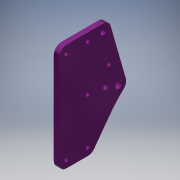
# Autodesk Inventor part: carriage plate square 2
Saved by Autodesk Inventor 2017 SP1 (Build 210196100, 196)
## iProperties
Created: 2018-01-19
Part Number: carriage plate square 2
Material: Aluminum 6061
Document SubType Name: Modeling
Designer: Ben
Density: 2.7 g/cm^3
Appearance: Smooth - Purple
Mass: 147.998 g
Surface Area: 209.147 cm^2
Volume: 54.8139 cm^3
Author: Ben
Autodesk Inventor part; units mm, degrees
ref_plane "YZ Plane" through (0, 0, 0) normal (1, 0, 0) x (0, 1, 0)
ref_plane "XZ Plane" through (0, 0, 0) normal (0, 1, 0) x (-1, 0, 0)
ref_plane "XY Plane" through (0, 0, 0) normal (0, 0, 1) x (1, 0, 0)
sketch "Sketch1" plane through (0, 0, 0) normal (1, 0, 0) x (0, 1, 0)
  line L0 (-420.7503, 12.7) -> (420.7488, 12.7) construction
  line L1 (420.7488, 12.7) -> (420.7488, -12.7) construction
  line L2 (420.7488, -12.7) -> (-420.7503, -12.7) construction
  line L3 (-420.7503, -12.7) -> (-420.7503, 12.7) construction
  line L4 (0, 0) -> (0, -26.6192) construction
  circle A0 centre (0, -26.6192) radius 2.54
  circle A1 centre (38.1, 26.6192) radius 2.54
  circle A2 centre (-76.2, 26.6192) radius 2.54
  line L5 (38.1, 26.6192) -> (-76.2, 26.6192) construction
  line L6 (0, 0) -> (0, 26.6192) construction
  circle A3 centre (0, -26.6192) radius 15.875 construction
  circle A4 centre (38.1, 26.6192) radius 15.875 construction
  circle A5 centre (-76.2, 26.6192) radius 15.875 construction
  line L7 (0, -26.6192) -> (-76.2, 26.6192) construction
  arc A6 (47.625, 26.6192) -> (38.1, 36.1442) centre (38.1, 26.6192) ccw
  arc A7 (-76.2, 36.1442) -> (-85.725, 26.6192) centre (-76.2, 26.6192) ccw
  line L8 (38.1, 36.1442) -> (-76.2, 36.1442)
  line L9 (47.625, 26.6192) -> (47.625, -19.05)
  line L10 (-85.725, 0) -> (-85.725, 26.6192)
  line L11 (-76.2, 26.6192) -> (-76.2, 0) construction
  line L12 (38.1, 26.6192) -> (38.1, 0) construction
  circle A8 centre (38.1, 0) radius 2.667
  circle A9 centre (-76.2, 0) radius 2.667
  line L13 (47.625, 0) -> (-85.725, 0) construction
  line L14 (-85.725, 0) -> (-420.7503, 0) construction
  circle A10 centre (-19.05, 0) radius 2.667
  line L15 (0, -26.6192) -> (38.1, 26.6192) construction
  line L16 (0, -26.6192) -> (0, -52.0192) construction
  line L17 (13.9446, -26.6192) -> (-16.4809, -26.6192) construction
  circle A11 centre (38.1, -19.05) radius 3.302
  circle A12 centre (-22.225, -22.225) radius 3.302
  line L18 (38.1, -19.05) -> (38.1, 0) construction
  arc A13 (40.7167, -28.2085) -> (47.625, -19.05) centre (38.1, -19.05) ccw
  line L19 (-25.9583, -47.2585) -> (40.7167, -28.2085)
  arc A14 (-85.725, 0) -> (-81.8213, -7.6894) centre (-76.2, 0) ccw
  circle A15 centre (-28.575, -38.1) radius 4.064
  arc A16 (-35.49, -44.6504) -> (-25.9583, -47.2585) centre (-28.575, -38.1) ccw
  circle A17 centre (-28.575, -38.1) radius 9.525 construction
  line L20 (-28.575, -12.7) -> (-28.575, -28.575) construction
  line L21 (-28.575, -47.625) -> (133.2586, -47.625) construction
  line L22 (-28.575, -47.625) -> (-28.575, -47.625) construction
  arc A18 (-35.49, -44.6504) -> (-56.1899, -26.427) centre (-146.1302, -149.4575) ccw
  line L23 (-56.1899, -26.427) -> (-81.8213, -7.6894)
  circle A19 centre (-28.575, -38.1) radius 14.2875 construction
  point P0 (0, -42.4942)
  dimension "d3" = 31.75
  dimension "d0" = 25.4
  dimension "d1" = 5.08
  dimension "d2" = 13.9192
  dimension "d4" = 38.1
  dimension "d5" = 76.2
  dimension "d6" = 9.525
  dimension "d9" = 5.334
  dimension "d10" = 25.4
  dimension "d14" = 6.35
  dimension "d15" = 9.525
  dimension "d17" = 3.175
  dimension "d18" = 22.225
  dimension "d19" = 8.128
  dimension "d20" = 6.604
  dimension "d26" = 19.05
  dimension "d27" = 12.7139
  dimension "d28" = 0
  dimension "d29" = 34.925
  dimension "d31" = 28.575
  dimension "d32" = 152.4
  dimension "d33" = 31.75
  dimension "d34" = 34.925
  dimension "d35" = 28.575
  constraints: 48 end point, 19 centre point, 15 coincident, 15 point on circle, 11 tangent, 10 point on line, 8 vertical, 7 equal radius, 5 horizontal, 4 perpendicular, 2 collinear, 2 midpoint, 2 parallel, 1 vertical alignment, 4 other
  measures "d0" distance of L0.end L1.end
  measures "d1" diameter of A0
  measures "d2" distance from line of L2 L4.end
  measures "d4" horizontal distance of L5.start L4.end
  measures "d5" distance from line of A2.centre L6
  measures "d6" radius of A6
  measures "d9" diameter of A8
  measures "d10" distance of L15.start L16.end
  measures "d14" distance from line of L2 L18.start
  measures "d15" distance from line of L2 A12.centre
  measures "d17" vertical distance of A12.centre L18.start
  measures "d18" horizontal distance of A12.centre L4.end
  measures "d19" diameter of A15
  measures "d20" diameter of A12
  measures "d26" diameter of A17
  measures "d27" distance from line of L4.end L19
  measures "d28" distance of L21.start L22.end
  measures "d29" distance between parallel lines of L2 L21
  measures "d31" distance from line of A15.centre L4
  measures "d32" radius of A18
  measures "d33" distance of L23.start L23.end
  measures "d34" distance from line of L2 L21.start
  measures "d35" diameter of A19
extrude "Extrusion1" add sketch "Sketch1" along normal blind 6.35
body "Solid1"
